Autodesk Fusion 360 part; units mm, degrees
note: some values were not read from the file. Set by a fixed rule: which sketch regions a step uses.
(part 5 of 6)
  spline S21 degree 5 poles (-7.8946, -5.2845) (-7.8923, -5.2844) (-7.8878, -5.2843) (-7.8811, -5.2842) (-7.8721, -5.284) (-7.8608, -5.2837) (-7.8496, -5.2835) (-7.8385, -5.2832) (-7.8273, -5.2828) (-7.8162, -5.2825) (-7.8052, -5.2821) (-7.7941, -5.2817) (-7.7831, -5.2813) (-7.7721, -5.2808) (-7.7611, -5.2803) (-7.7502, -5.2798) (-7.7393, -5.2793) (-7.7284, -5.2788) (-7.7175, -5.2782) (-7.7067, -5.2776) (-7.6959, -5.277) (-7.6852, -5.2764) (-7.6744, -5.2757) (-7.6637, -5.275) (-7.6531, -5.2743) (-7.6424, -5.2736) (-7.6318, -5.2729) (-7.6212, -5.2721) (-7.6107, -5.2713) (-7.6002, -5.2705) (-7.5897, -5.2697) (-7.5792, -5.2688) (-7.5688, -5.2679) (-7.5584, -5.2671) (-7.5481, -5.2661) (-7.5377, -5.2652) (-7.5274, -5.2642) (-7.5172, -5.2633) (-7.5069, -5.2623) (-7.4967, -5.2613) (-7.4865, -5.2602) (-7.4764, -5.2592) (-7.4663, -5.2581) (-7.4562, -5.257) (-7.4462, -5.2559) (-7.4362, -5.2547) (-7.4262, -5.2536) (-7.4163, -5.2524) (-7.4064, -5.2512) (-7.3965, -5.25) (-7.3866, -5.2487) (-7.3768, -5.2475) (-7.3671, -5.2462) (-7.3573, -5.2449) (-7.3476, -5.2436) (-7.3379, -5.2423) (-7.3283, -5.2409) (-7.3187, -5.2396) (-7.3091, -5.2382) (-7.2996, -5.2368) (-7.2901, -5.2354) (-7.2806, -5.2339) (-7.2712, -5.2325) (-7.2618, -5.231) (-7.2524, -5.2295) (-7.2431, -5.228) (-7.2338, -5.2265) (-7.2246, -5.225) (-7.2154, -5.2234) (-7.2062, -5.2219) (-7.197, -5.2203) (-7.1879, -5.2187) (-7.1789, -5.2171) (-7.1698, -5.2154) (-7.1608, -5.2138) (-7.1519, -5.2121) (-7.1429, -5.2104) (-7.1341, -5.2087) (-7.1252, -5.207) (-7.1164, -5.2053) (-7.1076, -5.2036) (-7.0989, -5.2018) (-7.0902, -5.2001) (-7.0815, -5.1983) (-7.0729, -5.1965) (-7.0643, -5.1947) (-7.0558, -5.1929) (-7.0473, -5.191) (-7.0388, -5.1892) (-7.0304, -5.1873) (-7.022, -5.1854) (-7.0136, -5.1836) (-7.0053, -5.1817) (-6.997, -5.1797) (-6.9888, -5.1778) (-6.9806, -5.1759) (-6.9725, -5.1739) (-6.9644, -5.172) (-6.9563, -5.17) (-6.9483, -5.168) (-6.9403, -5.166) (-6.9323, -5.164) (-6.9244, -5.162) (-6.9165, -5.16) (-6.9087, -5.158) (-6.9009, -5.1559) (-6.8932, -5.1539) (-6.8855, -5.1518) (-6.8778, -5.1498) (-6.8702, -5.1477) (-6.8626, -5.1456) (-6.8551, -5.1435) (-6.8476, -5.1414) (-6.8401, -5.1393) (-6.8327, -5.1371) (-6.8254, -5.135) (-6.818, -5.1329) (-6.8108, -5.1307) (-6.8035, -5.1286) (-6.7963, -5.1264) (-6.7892, -5.1242) (-6.7821, -5.1221) (-6.775, -5.1199) (-6.768, -5.1177) (-6.761, -5.1155) (-6.7541, -5.1133) (-6.7472, -5.1111) (-6.7404, -5.1089) (-6.7336, -5.1067) (-6.7269, -5.1045) (-6.7201, -5.1023) (-6.7135, -5.1) (-6.7069, -5.0978) (-6.7003, -5.0956) (-6.6938, -5.0933) (-6.6873, -5.0911) (-6.6809, -5.0889) (-6.6745, -5.0866) (-6.6682, -5.0844) (-6.6619, -5.0821) (-6.6556, -5.0799) (-6.6495, -5.0776) (-6.6433, -5.0754) (-6.6372, -5.0731) (-6.6312, -5.0709) (-6.6252, -5.0686) (-6.6192, -5.0664) (-6.6133, -5.0641) (-6.6074, -5.0618) (-6.6016, -5.0596) (-6.5959, -5.0573) (-6.5901, -5.0551) (-6.5845, -5.0528) (-6.5789, -5.0506) (-6.5733, -5.0483) (-6.5678, -5.0461) (-6.5623, -5.0439) (-6.5569, -5.0416) (-6.5515, -5.0394) (-6.5462, -5.0372) (-6.541, -5.0349) (-6.5357, -5.0327) (-6.5306, -5.0305) (-6.5255, -5.0283) (-6.5204, -5.0261) (-6.5154, -5.0239) (-6.5104, -5.0217) (-6.5055, -5.0195) (-6.5007, -5.0174) (-6.4959, -5.0152) (-6.4911, -5.013) (-6.4864, -5.0109) (-6.4818, -5.0087) (-6.4772, -5.0066) (-6.4727, -5.0045) (-6.4682, -5.0023) (-6.4637, -5.0002) (-6.4594, -4.9981) (-6.455, -4.9961) (-6.4508, -4.994) (-6.4466, -4.9919) (-6.4424, -4.9899) (-6.4383, -4.9878) (-6.4343, -4.9858) (-6.4303, -4.9838) (-6.4263, -4.9818) (-6.4224, -4.9798) (-6.4186, -4.9778) (-6.4149, -4.9759) (-6.4111, -4.9739) (-6.4075, -4.972) (-6.4039, -4.9701) (-6.4003, -4.9682) (-6.3969, -4.9664) (-6.3934, -4.9645) (-6.3901, -4.9627) (-6.3868, -4.9608) (-6.3835, -4.9591) (-6.3803, -4.9573) (-6.3772, -4.9555) (-6.3741, -4.9538) (-6.3711, -4.9521) (-6.3681, -4.9504) (-6.3652, -4.9487) (-6.3624, -4.9471) (-6.3596, -4.9454) (-6.3569, -4.9439) (-6.3543, -4.9423) (-6.3517, -4.9407) (-6.3491, -4.9392) (-6.3467, -4.9377) (-6.3443, -4.9363) (-6.3419, -4.9348) (-6.3396, -4.9334) (-6.3374, -4.932) (-6.3353, -4.9307) (-6.3332, -4.9294) (-6.3311, -4.9281) (-6.3292, -4.9268) (-6.3273, -4.9256) (-6.3254, -4.9244) (-6.3237, -4.9233) (-6.322, -4.9221) (-6.3203, -4.9211) (-6.3188, -4.92) (-6.3173, -4.919) (-6.3158, -4.918) (-6.3144, -4.9171) (-6.3131, -4.9162) (-6.3119, -4.9153) (-6.3107, -4.9145) (-6.3096, -4.9138) (-6.3086, -4.913) (-6.3076, -4.9124) (-6.3067, -4.9117) (-6.3059, -4.9111) (-6.3052, -4.9106) (-6.3045, -4.9101) (-6.3039, -4.9096) (-6.3033, -4.9092) (-6.3029, -4.9089) (-6.3026, -4.9086) (-6.3024, -4.9085) (-6.3022, -4.9084) (-6.3022, -4.9084) knots -1 -1 -1 -1 -1 -1 -0.99583333 -0.99166667 -0.9875 -0.98333333 -0.97916667 -0.975 -0.97083333 -0.96666667 -0.9625 -0.95833333 -0.95416667 -0.95 -0.94583333 -0.94166667 -0.9375 -0.93333333 -0.92916667 -0.925 -0.92083333 -0.91666667 -0.9125 -0.90833333 -0.90416667 -0.9 -0.89583333 -0.89166667 -0.8875 -0.88333333 -0.87916667 -0.875 -0.87083333 -0.86666667 -0.8625 -0.85833333 -0.85416667 -0.85 -0.84583333 -0.84166667 -0.8375 -0.83333333 -0.82916667 -0.825 -0.82083333 -0.81666667 -0.8125 -0.80833333 -0.80416667 -0.8 -0.79583333 -0.79166667 -0.7875 -0.78333333 -0.77916667 -0.775 -0.77083333 -0.76666667 -0.7625 -0.75833333 -0.75416667 -0.75 -0.74583333 -0.74166667 -0.7375 -0.73333333 -0.72916667 -0.725 -0.72083333 -0.71666667 -0.7125 -0.70833333 -0.70416667 -0.7 -0.69583333 -0.69166667 -0.6875 -0.68333333 -0.67916667 -0.675 -0.67083333 -0.66666667 -0.6625 -0.65833333 -0.65416667 -0.65 -0.64583333 -0.64166667 -0.6375 -0.63333333 -0.62916667 -0.625 -0.62083333 -0.61666667 -0.6125 -0.60833333 -0.60416667 -0.6 -0.59583333 -0.59166667 -0.5875 -0.58333333 -0.57916667 -0.575 -0.57083333 -0.56666667 -0.5625 -0.55833333 -0.55416667 -0.55 -0.54583333 -0.54166667 -0.5375 -0.53333333 -0.52916667 -0.525 -0.52083333 -0.51666667 -0.5125 -0.50833333 -0.50416667 -0.5 -0.49583333 -0.49166667 -0.4875 -0.48333333 -0.47916667 -0.475 -0.47083333 -0.46666667 -0.4625 -0.45833333 -0.45416667 -0.45 -0.44583333 -0.44166667 -0.4375 -0.43333333 -0.42916667 -0.425 -0.42083333 -0.41666667 -0.4125 -0.40833333 -0.40416667 -0.4 -0.39583333 -0.39166667 -0.3875 -0.38333333 -0.37916667 -0.375 -0.37083333 -0.36666667 -0.3625 -0.35833333 -0.35416667 -0.35 -0.34583333 -0.34166667 -0.3375 -0.33333333 -0.32916667 -0.325 -0.32083333 -0.31666667 -0.3125 -0.30833333 -0.30416667 -0.3 -0.29583333 -0.29166667 -0.2875 -0.28333333 -0.27916667 -0.275 -0.27083333 -0.26666667 -0.2625 -0.25833333 -0.25416667 -0.25 -0.24583333 -0.24166667 -0.2375 -0.23333333 -0.22916667 -0.225 -0.22083333 -0.21666667 -0.2125 -0.20833333 -0.20416667 -0.2 -0.19583333 -0.19166667 -0.1875 -0.18333333 -0.17916667 -0.175 -0.17083333 -0.16666667 -0.1625 -0.15833333 -0.15416667 -0.15 -0.14583333 -0.14166667 -0.1375 -0.13333333 -0.12916667 -0.125 -0.12083333 -0.11666667 -0.1125 -0.10833333 -0.10416667 -0.1 -0.09583333 -0.09166667 -0.0875 -0.08333333 -0.07916667 -0.075 -0.07083333 -0.06666667 -0.0625 -0.05833333 -0.05416667 -0.05 -0.04583333 -0.04166667 -0.0375 -0.03333333 -0.02916667 -0.025 -0.02083333 -0.01666667 -0.0125 -0.00833333 -0.00416667 0 0 0 0 0 0
  line L42 (-6.3022, -4.9084) -> (-6.3016, -4.9079)
  line L43 (-6.3016, -4.9079) -> (-5.7199, -4.4548)
  arc A22 (-5.7199, -4.4548) -> (-4.9636, -5.2844) centre (0, 0) ccw
  line L44 (-4.9636, -5.2844) -> (-5.4684, -5.8219)
  line L45 (-5.4684, -5.8219) -> (-5.4689, -5.8224)
  spline S22 degree 5 poles (-5.4689, -5.8224) (-5.469, -5.8225) (-5.4691, -5.8226) (-5.4692, -5.8228) (-5.4695, -5.823) (-5.4699, -5.8235) (-5.4703, -5.824) (-5.4708, -5.8245) (-5.4714, -5.8252) (-5.472, -5.8259) (-5.4727, -5.8266) (-5.4734, -5.8275) (-5.4742, -5.8284) (-5.475, -5.8293) (-5.4758, -5.8304) (-5.4768, -5.8314) (-5.4777, -5.8326) (-5.4787, -5.8338) (-5.4798, -5.8351) (-5.4809, -5.8364) (-5.482, -5.8378) (-5.4832, -5.8393) (-5.4845, -5.8408) (-5.4857, -5.8424) (-5.487, -5.8441) (-5.4884, -5.8458) (-5.4898, -5.8476) (-5.4912, -5.8494) (-5.4927, -5.8513) (-5.4942, -5.8533) (-5.4957, -5.8553) (-5.4973, -5.8574) (-5.4989, -5.8595) (-5.5006, -5.8617) (-5.5023, -5.864) (-5.504, -5.8663) (-5.5057, -5.8687) (-5.5075, -5.8711) (-5.5093, -5.8736) (-5.5111, -5.8762) (-5.513, -5.8788) (-5.5149, -5.8815) (-5.5168, -5.8842) (-5.5188, -5.887) (-5.5208, -5.8898) (-5.5228, -5.8927) (-5.5248, -5.8957) (-5.5269, -5.8987) (-5.529, -5.9018) (-5.5311, -5.9049) (-5.5332, -5.9081) (-5.5354, -5.9113) (-5.5376, -5.9146) (-5.5398, -5.918) (-5.542, -5.9214) (-5.5443, -5.9249) (-5.5465, -5.9284) (-5.5488, -5.9319) (-5.5511, -5.9356) (-5.5535, -5.9393) (-5.5558, -5.943) (-5.5582, -5.9468) (-5.5606, -5.9506) (-5.563, -5.9545) (-5.5654, -5.9585) (-5.5679, -5.9625) (-5.5703, -5.9665) (-5.5728, -5.9706) (-5.5753, -5.9748) (-5.5778, -5.979) (-5.5803, -5.9833) (-5.5829, -5.9876) (-5.5854, -5.992) (-5.588, -5.9964) (-5.5906, -6.0009) (-5.5932, -6.0054) (-5.5958, -6.01) (-5.5984, -6.0146) (-5.601, -6.0193) (-5.6036, -6.0241) (-5.6063, -6.0288) (-5.6089, -6.0337) (-5.6116, -6.0386) (-5.6143, -6.0435) (-5.617, -6.0485) (-5.6197, -6.0535) (-5.6224, -6.0586) (-5.6251, -6.0637) (-5.6278, -6.0689) (-5.6306, -6.0742) (-5.6333, -6.0795) (-5.6361, -6.0848) (-5.6388, -6.0902) (-5.6416, -6.0956) (-5.6444, -6.1011) (-5.6471, -6.1066) (-5.6499, -6.1122) (-5.6527, -6.1178) (-5.6555, -6.1235) (-5.6583, -6.1292) (-5.6611, -6.135) (-5.6639, -6.1408) (-5.6667, -6.1467) (-5.6695, -6.1526) (-5.6723, -6.1585) (-5.6751, -6.1645) (-5.6779, -6.1706) (-5.6808, -6.1767) (-5.6836, -6.1829) (-5.6864, -6.189) (-5.6892, -6.1953) (-5.6921, -6.2016) (-5.6949, -6.2079) (-5.6977, -6.2143) (-5.7006, -6.2207) (-5.7034, -6.2272) (-5.7062, -6.2337) (-5.709, -6.2402) (-5.7119, -6.2469) (-5.7147, -6.2535) (-5.7175, -6.2602) (-5.7204, -6.2669) (-5.7232, -6.2737) (-5.726, -6.2806) (-5.7288, -6.2874) (-5.7316, -6.2943) (-5.7344, -6.3013) (-5.7373, -6.3083) (-5.7401, -6.3154) (-5.7429, -6.3225) (-5.7457, -6.3296) (-5.7485, -6.3368) (-5.7513, -6.344) (-5.7541, -6.3513) (-5.7568, -6.3586) (-5.7596, -6.3659) (-5.7624, -6.3733) (-5.7652, -6.3808) (-5.7679, -6.3882) (-5.7707, -6.3958) (-5.7734, -6.4033) (-5.7762, -6.4109) (-5.7789, -6.4186) (-5.7817, -6.4263) (-5.7844, -6.434) (-5.7871, -6.4418) (-5.7898, -6.4496) (-5.7925, -6.4574) (-5.7952, -6.4653) (-5.7979, -6.4733) (-5.8006, -6.4813) (-5.8033, -6.4893) (-5.8059, -6.4973) (-5.8086, -6.5054) (-5.8112, -6.5136) (-5.8139, -6.5218) (-5.8165, -6.53) (-5.8191, -6.5382) (-5.8217, -6.5465) (-5.8243, -6.5549) (-5.8269, -6.5633) (-5.8295, -6.5717) (-5.8321, -6.5801) (-5.8346, -6.5886) (-5.8372, -6.5972) (-5.8397, -6.6057) (-5.8423, -6.6144) (-5.8448, -6.623) (-5.8473, -6.6317) (-5.8498, -6.6404) (-5.8523, -6.6492) (-5.8547, -6.658) (-5.8572, -6.6669) (-5.8596, -6.6757) (-5.8621, -6.6847) (-5.8645, -6.6936) (-5.8669, -6.7026) (-5.8693, -6.7117) (-5.8717, -6.7207) (-5.874, -6.7298) (-5.8764, -6.739) (-5.8787, -6.7482) (-5.8811, -6.7574) (-5.8834, -6.7666) (-5.8857, -6.7759) (-5.888, -6.7853) (-5.8902, -6.7946) (-5.8925, -6.804) (-5.8948, -6.8135) (-5.897, -6.8229) (-5.8992, -6.8324) (-5.9014, -6.842) (-5.9036, -6.8516) (-5.9057, -6.8612) (-5.9079, -6.8708) (-5.91, -6.8805) (-5.9122, -6.8902) (-5.9143, -6.9) (-5.9164, -6.9098) (-5.9184, -6.9196) (-5.9205, -6.9295) (-5.9225, -6.9394) (-5.9245, -6.9493) (-5.9266, -6.9593) (-5.9285, -6.9693) (-5.9305, -6.9793) (-5.9325, -6.9894) (-5.9344, -6.9995) (-5.9363, -7.0096) (-5.9382, -7.0198) (-5.9401, -7.03) (-5.942, -7.0402) (-5.9438, -7.0505) (-5.9457, -7.0608) (-5.9475, -7.0711) (-5.9493, -7.0815) (-5.9511, -7.0919) (-5.9528, -7.1023) (-5.9546, -7.1128) (-5.9563, -7.1232) (-5.958, -7.1338) (-5.9597, -7.1443) (-5.9613, -7.1549) (-5.963, -7.1656) (-5.9646, -7.1762) (-5.9662, -7.1869) (-5.9678, -7.1976) (-5.9693, -7.2084) (-5.9709, -7.2191) (-5.9724, -7.23) (-5.9739, -7.2408) (-5.9754, -7.2517) (-5.9769, -7.2626) (-5.9783, -7.2735) (-5.9797, -7.2845) (-5.9811, -7.2955) (-5.9825, -7.3065) (-5.9839, -7.3176) (-5.9852, -7.3287) (-5.9865, -7.3398) (-5.9878, -7.3509) (-5.9888, -7.3599) (-5.9896, -7.3666) (-5.9901, -7.3711) (-5.9903, -7.3733) knots 0 0 0 0 0 0 0.00416667 0.00833333 0.0125 0.01666667 0.02083333 0.025 0.02916667 0.03333333 0.0375 0.04166667 0.04583333 0.05 0.05416667 0.05833333 0.0625 0.06666667 0.07083333 0.075 0.07916667 0.08333333 0.0875 0.09166667 0.09583333 0.1 0.10416667 0.10833333 0.1125 0.11666667 0.12083333 0.125 0.12916667 0.13333333 0.1375 0.14166667 0.14583333 0.15 0.15416667 0.15833333 0.1625 0.16666667 0.17083333 0.175 0.17916667 0.18333333 0.1875 0.19166667 0.19583333 0.2 0.20416667 0.20833333 0.2125 0.21666667 0.22083333 0.225 0.22916667 0.23333333 0.2375 0.24166667 0.24583333 0.25 0.25416667 0.25833333 0.2625 0.26666667 0.27083333 0.275 0.27916667 0.28333333 0.2875 0.29166667 0.29583333 0.3 0.30416667 0.30833333 0.3125 0.31666667 0.32083333 0.325 0.32916667 0.33333333 0.3375 0.34166667 0.34583333 0.35 0.35416667 0.35833333 0.3625 0.36666667 0.37083333 0.375 0.37916667 0.38333333 0.3875 0.39166667 0.39583333 0.4 0.40416667 0.40833333 0.4125 0.41666667 0.42083333 0.425 0.42916667 0.43333333 0.4375 0.44166667 0.44583333 0.45 0.45416667 0.45833333 0.4625 0.46666667 0.47083333 0.475 0.47916667 0.48333333 0.4875 0.49166667 0.49583333 0.5 0.50416667 0.50833333 0.5125 0.51666667 0.52083333 0.525 0.52916667 0.53333333 0.5375 0.54166667 0.54583333 0.55 0.55416667 0.55833333 0.5625 0.56666667 0.57083333 0.575 0.57916667 0.58333333 0.5875 0.59166667 0.59583333 0.6 0.60416667 0.60833333 0.6125 0.61666667 0.62083333 0.625 0.62916667 0.63333333 0.6375 0.64166667 0.64583333 0.65 0.65416667 0.65833333 0.6625 0.66666667 0.67083333 0.675 0.67916667 0.68333333 0.6875 0.69166667 0.69583333 0.7 0.70416667 0.70833333 0.7125 0.71666667 0.72083333 0.725 0.72916667 0.73333333 0.7375 0.74166667 0.74583333 0.75 0.75416667 0.75833333 0.7625 0.76666667 0.77083333 0.775 0.77916667 0.78333333 0.7875 0.79166667 0.79583333 0.8 0.80416667 0.80833333 0.8125 0.81666667 0.82083333 0.825 0.82916667 0.83333333 0.8375 0.84166667 0.84583333 0.85 0.85416667 0.85833333 0.8625 0.86666667 0.87083333 0.875 0.87916667 0.88333333 0.8875 0.89166667 0.89583333 0.9 0.90416667 0.90833333 0.9125 0.91666667 0.92083333 0.925 0.92916667 0.93333333 0.9375 0.94166667 0.94583333 0.95 0.95416667 0.95833333 0.9625 0.96666667 0.97083333 0.975 0.97916667 0.98333333 0.9875 0.99166667 0.99583333 1 1 1 1 1 1
  arc A23 (-5.9903, -7.3733) -> (-5.4525, -7.7795) centre (0, 0) ccw
  spline S23 degree 5 poles (-5.4525, -7.7795) (-5.4504, -7.7786) (-5.4463, -7.7769) (-5.44, -7.7743) (-5.4317, -7.7709) (-5.4213, -7.7666) (-5.411, -7.7623) (-5.4007, -7.758) (-5.3904, -7.7536) (-5.3802, -7.7493) (-5.37, -7.7449) (-5.3598, -7.7406) (-5.3497, -7.7362) (-5.3396, -7.7318) (-5.3296, -7.7274) (-5.3195, -7.723) (-5.3096, -7.7186) (-5.2996, -7.7141) (-5.2897, -7.7097) (-5.2798, -7.7052) (-5.27, -7.7008) (-5.2602, -7.6963) (-5.2504, -7.6918) (-5.2407, -7.6873) (-5.231, -7.6828) (-5.2213, -7.6783) (-5.2117, -7.6737) (-5.2021, -7.6692) (-5.1925, -7.6647) (-5.183, -7.6601) (-5.1736, -7.6555) (-5.1641, -7.651) (-5.1547, -7.6464) (-5.1453, -7.6418) (-5.136, -7.6372) (-5.1267, -7.6326) (-5.1175, -7.628) (-5.1082, -7.6234) (-5.099, -7.6187) (-5.0899, -7.6141) (-5.0808, -7.6095) (-5.0717, -7.6048) (-5.0627, -7.6001) (-5.0537, -7.5955) (-5.0447, -7.5908) (-5.0358, -7.5861) (-5.0269, -7.5815) (-5.0181, -7.5768) (-5.0093, -7.5721) (-5.0005, -7.5674) (-4.9918, -7.5627) (-4.9831, -7.5579) (-4.9744, -7.5532) (-4.9658, -7.5485) (-4.9572, -7.5438) (-4.9487, -7.5391) (-4.9402, -7.5343) (-4.9317, -7.5296) (-4.9233, -7.5248) (-4.9149, -7.5201) (-4.9066, -7.5153) (-4.8983, -7.5106) (-4.89, -7.5058) (-4.8818, -7.501) (-4.8736, -7.4963) (-4.8654, -7.4915) (-4.8573, -7.4867) (-4.8492, -7.482) (-4.8412, -7.4772) (-4.8332, -7.4724) (-4.8253, -7.4676) (-4.8173, -7.4628) (-4.8095, -7.4581) (-4.8016, -7.4533) (-4.7938, -7.4485) (-4.7861, -7.4437) (-4.7784, -7.4389) (-4.7707, -7.4341) (-4.7631, -7.4293) (-4.7555, -7.4245) (-4.7479, -7.4198) (-4.7404, -7.415) (-4.7329, -7.4102) (-4.7255, -7.4054) (-4.7181, -7.4006) (-4.7107, -7.3958) (-4.7034, -7.391) (-4.6962, -7.3862) (-4.6889, -7.3815) (-4.6817, -7.3767) (-4.6746, -7.3719) (-4.6675, -7.3671) (-4.6604, -7.3624) (-4.6534, -7.3576) (-4.6464, -7.3528) (-4.6395, -7.3481) (-4.6326, -7.3433) (-4.6257, -7.3386) (-4.6189, -7.3338) (-4.6121, -7.3291) (-4.6054, -7.3243) (-4.5987, -7.3196) (-4.5921, -7.3148) (-4.5855, -7.3101) (-4.5789, -7.3054) (-4.5724, -7.3007) (-4.5659, -7.296) (-4.5595, -7.2913) (-4.5531, -7.2866) (-4.5467, -7.2819) (-4.5404, -7.2772) (-4.5341, -7.2725) (-4.5279, -7.2678) (-4.5217, -7.2632) (-4.5156, -7.2585) (-4.5095, -7.2539) (-4.5034, -7.2492) (-4.4974, -7.2446) (-4.4914, -7.24) (-4.4855, -7.2354) (-4.4796, -7.2308) (-4.4738, -7.2262) (-4.468, -7.2216) (-4.4623, -7.217) (-4.4565, -7.2124) (-4.4509, -7.2079) (-4.4453, -7.2034) (-4.4397, -7.1988) (-4.4341, -7.1943) (-4.4286, -7.1898) (-4.4232, -7.1853) (-4.4178, -7.1808) (-4.4124, -7.1764) (-4.4071, -7.1719) (-4.4018, -7.1675) (-4.3966, -7.1631) (-4.3914, -7.1586) (-4.3863, -7.1542) (-4.3812, -7.1499) (-4.3762, -7.1455) (-4.3711, -7.1411) (-4.3662, -7.1368) (-4.3613, -7.1325) (-4.3564, -7.1282) (-4.3516, -7.1239) (-4.3468, -7.1196) (-4.342, -7.1154) (-4.3373, -7.1111) (-4.3327, -7.1069) (-4.3281, -7.1027) (-4.3235, -7.0985) (-4.319, -7.0944) (-4.3145, -7.0902) (-4.3101, -7.0861) (-4.3057, -7.082) (-4.3014, -7.0779) (-4.2971, -7.0738) (-4.2929, -7.0698) (-4.2887, -7.0658) (-4.2845, -7.0618) (-4.2804, -7.0578) (-4.2764, -7.0539) (-4.2724, -7.0499) (-4.2684, -7.046) (-4.2645, -7.0421) (-4.2606, -7.0383) (-4.2568, -7.0344) (-4.253, -7.0306) (-4.2492, -7.0269) (-4.2455, -7.0231) (-4.2419, -7.0194) (-4.2383, -7.0157) (-4.2347, -7.012) (-4.2312, -7.0083) (-4.2278, -7.0047) (-4.2243, -7.0011) (-4.221, -6.9976) (-4.2176, -6.994) (-4.2144, -6.9905) (-4.2111, -6.987) (-4.208, -6.9836) (-4.2048, -6.9802) (-4.2017, -6.9768) (-4.1987, -6.9734) (-4.1957, -6.9701) (-4.1927, -6.9668) (-4.1898, -6.9636) (-4.187, -6.9604) (-4.1842, -6.9572) (-4.1814, -6.954) (-4.1787, -6.9509) (-4.176, -6.9478) (-4.1734, -6.9448) (-4.1708, -6.9418) (-4.1683, -6.9388) (-4.1658, -6.9359) (-4.1634, -6.933) (-4.161, -6.9302) (-4.1587, -6.9274) (-4.1564, -6.9246) (-4.1542, -6.9219) (-4.152, -6.9192) (-4.1498, -6.9165) (-4.1477, -6.9139) (-4.1457, -6.9114) (-4.1437, -6.9089) (-4.1417, -6.9064) (-4.1398, -6.904) (-4.138, -6.9016) (-4.1361, -6.8993) (-4.1344, -6.897) (-4.1327, -6.8947) (-4.131, -6.8925) (-4.1294, -6.8904) (-4.1278, -6.8883) (-4.1263, -6.8863) (-4.1248, -6.8843) (-4.1234, -6.8824) (-4.122, -6.8805) (-4.1207, -6.8787) (-4.1194, -6.8769) (-4.1182, -6.8752) (-4.117, -6.8735) (-4.1158, -6.8719) (-4.1148, -6.8704) (-4.1137, -6.8689) (-4.1127, -6.8675) (-4.1118, -6.8661) (-4.1109, -6.8648) (-4.11, -6.8635) (-4.1092, -6.8624) (-4.1085, -6.8612) (-4.1078, -6.8602) (-4.1072, -6.8592) (-4.1065, -6.8583) (-4.106, -6.8574) (-4.1055, -6.8567) (-4.105, -6.856) (-4.1046, -6.8553) (-4.1043, -6.8548) (-4.104, -6.8543) (-4.1037, -6.8539) (-4.1036, -6.8537) (-4.1035, -6.8536) (-4.1035, -6.8535) knots -1 -1 -1 -1 -1 -1 -0.99583333 -0.99166667 -0.9875 -0.98333333 -0.97916667 -0.975 -0.97083333 -0.96666667 -0.9625 -0.95833333 -0.95416667 -0.95 -0.94583333 -0.94166667 -0.9375 -0.93333333 -0.92916667 -0.925 -0.92083333 -0.91666667 -0.9125 -0.90833333 -0.90416667 -0.9 -0.89583333 -0.89166667 -0.8875 -0.88333333 -0.87916667 -0.875 -0.87083333 -0.86666667 -0.8625 -0.85833333 -0.85416667 -0.85 -0.84583333 -0.84166667 -0.8375 -0.83333333 -0.82916667 -0.825 -0.82083333 -0.81666667 -0.8125 -0.80833333 -0.80416667 -0.8 -0.79583333 -0.79166667 -0.7875 -0.78333333 -0.77916667 -0.775 -0.77083333 -0.76666667 -0.7625 -0.75833333 -0.75416667 -0.75 -0.74583333 -0.74166667 -0.7375 -0.73333333 -0.72916667 -0.725 -0.72083333 -0.71666667 -0.7125 -0.70833333 -0.70416667 -0.7 -0.69583333 -0.69166667 -0.6875 -0.68333333 -0.67916667 -0.675 -0.67083333 -0.66666667 -0.6625 -0.65833333 -0.65416667 -0.65 -0.64583333 -0.64166667 -0.6375 -0.63333333 -0.62916667 -0.625 -0.62083333 -0.61666667 -0.6125 -0.60833333 -0.60416667 -0.6 -0.59583333 -0.59166667 -0.5875 -0.58333333 -0.57916667 -0.575 -0.57083333 -0.56666667 -0.5625 -0.55833333 -0.55416667 -0.55 -0.54583333 -0.54166667 -0.5375 -0.53333333 -0.52916667 -0.525 -0.52083333 -0.51666667 -0.5125 -0.50833333 -0.50416667 -0.5 -0.49583333 -0.49166667 -0.4875 -0.48333333 -0.47916667 -0.475 -0.47083333 -0.46666667 -0.4625 -0.45833333 -0.45416667 -0.45 -0.44583333 -0.44166667 -0.4375 -0.43333333 -0.42916667 -0.425 -0.42083333 -0.41666667 -0.4125 -0.40833333 -0.40416667 -0.4 -0.39583333 -0.39166667 -0.3875 -0.38333333 -0.37916667 -0.375 -0.37083333 -0.36666667 -0.3625 -0.35833333 -0.35416667 -0.35 -0.34583333 -0.34166667 -0.3375 -0.33333333 -0.32916667 -0.325 -0.32083333 -0.31666667 -0.3125 -0.30833333 -0.30416667 -0.3 -0.29583333 -0.29166667 -0.2875 -0.28333333 -0.27916667 -0.275 -0.27083333 -0.26666667 -0.2625 -0.25833333 -0.25416667 -0.25 -0.24583333 -0.24166667 -0.2375 -0.23333333 -0.22916667 -0.225 -0.22083333 -0.21666667 -0.2125 -0.20833333 -0.20416667 -0.2 -0.19583333 -0.19166667 -0.1875 -0.18333333 -0.17916667 -0.175 -0.17083333 -0.16666667 -0.1625 -0.15833333 -0.15416667 -0.15 -0.14583333 -0.14166667 -0.1375 -0.13333333 -0.12916667 -0.125 -0.12083333 -0.11666667 -0.1125 -0.10833333 -0.10416667 -0.1 -0.09583333 -0.09166667 -0.0875 -0.08333333 -0.07916667 -0.075 -0.07083333 -0.06666667 -0.0625 -0.05833333 -0.05416667 -0.05 -0.04583333 -0.04166667 -0.0375 -0.03333333 -0.02916667 -0.025 -0.02083333 -0.01666667 -0.0125 -0.00833333 -0.00416667 0 0 0 0 0 0
  line L46 (-4.1035, -6.8535) -> (-4.1031, -6.8529)
  line L47 (-4.1031, -6.8529) -> (-3.7243, -6.2203)
  arc A24 (-3.7243, -6.2203) -> (-2.7195, -6.7206) centre (0, 0) ccw
  line L48 (-2.7195, -6.7206) -> (-2.9961, -7.4042)
  line L49 (-2.9961, -7.4042) -> (-2.9963, -7.4048)
  spline S24 degree 5 poles (-2.9963, -7.4048) (-2.9963, -7.4049) (-2.9964, -7.405) (-2.9965, -7.4053) (-2.9966, -7.4056) (-2.9968, -7.4062) (-2.9971, -7.4068) (-2.9973, -7.4075) (-2.9976, -7.4083) (-2.9979, -7.4092) (-2.9983, -7.4101) (-2.9987, -7.4112) (-2.9991, -7.4123) (-2.9995, -7.4135) (-2.9999, -7.4147) (-3.0004, -7.4161) (-3.0008, -7.4175) (-3.0014, -7.419) (-3.0019, -7.4206) (-3.0024, -7.4222) (-3.003, -7.424) (-3.0036, -7.4258) (-3.0041, -7.4276) (-3.0048, -7.4296) (-3.0054, -7.4316) (-3.006, -7.4337) (-3.0067, -7.4359) (-3.0074, -7.4381) (-3.008, -7.4404) (-3.0087, -7.4428) (-3.0094, -7.4452) (-3.0102, -7.4477) (-3.0109, -7.4503) (-3.0116, -7.4529) (-3.0124, -7.4557) (-3.0131, -7.4584) (-3.0139, -7.4613) (-3.0147, -7.4642) (-3.0155, -7.4672) (-3.0163, -7.4702) (-3.0171, -7.4734) (-3.0179, -7.4765) (-3.0187, -7.4798) (-3.0195, -7.4831) (-3.0203, -7.4864) (-3.0211, -7.4899) (-3.022, -7.4934) (-3.0228, -7.4969) (-3.0237, -7.5006) (-3.0245, -7.5042) (-3.0253, -7.508) (-3.0262, -7.5118) (-3.027, -7.5156) (-3.0279, -7.5196) (-3.0287, -7.5235) (-3.0296, -7.5276) (-3.0304, -7.5317) (-3.0313, -7.5358) (-3.0321, -7.5401) (-3.033, -7.5443) (-3.0338, -7.5487) (-3.0346, -7.5531) (-3.0355, -7.5575) (-3.0363, -7.562) (-3.0372, -7.5666) (-3.038, -7.5712) (-3.0388, -7.5759) (-3.0396, -7.5806) (-3.0405, -7.5854) (-3.0413, -7.5902) (-3.0421, -7.5951) (-3.0429, -7.6001) (-3.0437, -7.6051) (-3.0445, -7.6101) (-3.0453, -7.6152) (-3.0461, -7.6204) (-3.0468, -7.6256) (-3.0476, -7.6308) (-3.0483, -7.6362) (-3.0491, -7.6415) (-3.0498, -7.647) (-3.0506, -7.6524) (-3.0513, -7.6579) (-3.052, -7.6635) (-3.0527, -7.6691) (-3.0534, -7.6748) (-3.0541, -7.6805) (-3.0548, -7.6863) (-3.0555, -7.6921) (-3.0561, -7.698) (-3.0568, -7.7039) (-3.0574, -7.7099) (-3.058, -7.7159) (-3.0586, -7.722) (-3.0592, -7.7281) (-3.0598, -7.7342) (-3.0604, -7.7404) (-3.061, -7.7467) (-3.0615, -7.753) (-3.0621, -7.7593) (-3.0626, -7.7657) (-3.0631, -7.7722) (-3.0636, -7.7786) (-3.0641, -7.7852) (-3.0645, -7.7917) (-3.065, -7.7984) (-3.0654, -7.805) (-3.0659, -7.8117) (-3.0663, -7.8185) (-3.0667, -7.8253) (-3.0671, -7.8321) (-3.0674, -7.839) (-3.0678, -7.8459) (-3.0681, -7.8529) (-3.0684, -7.8599) (-3.0687, -7.867) (-3.069, -7.8741) (-3.0693, -7.8812) (-3.0695, -7.8884) (-3.0698, -7.8956) (-3.07, -7.9029) (-3.0702, -7.9102) (-3.0704, -7.9175) (-3.0705, -7.9249) (-3.0707, -7.9323) (-3.0708, -7.9398) (-3.0709, -7.9473) (-3.071, -7.9549) (-3.0711, -7.9624) (-3.0711, -7.9701) (-3.0712, -7.9777) (-3.0712, -7.9854) (-3.0712, -7.9932) (-3.0712, -8.001) (-3.0711, -8.0088) (-3.071, -8.0167) (-3.071, -8.0246) (-3.0709, -8.0325) (-3.0707, -8.0405) (-3.0706, -8.0485) (-3.0704, -8.0565) (-3.0702, -8.0646) (-3.07, -8.0727) (-3.0698, -8.0809) (-3.0695, -8.0891) (-3.0693, -8.0973) (-3.069, -8.1056) (-3.0687, -8.1139) (-3.0683, -8.1222) (-3.068, -8.1306) (-3.0676, -8.139) (-3.0672, -8.1474) (-3.0668, -8.1559) (-3.0663, -8.1644) (-3.0658, -8.173) (-3.0653, -8.1816) (-3.0648, -8.1902) (-3.0643, -8.1988) (-3.0637, -8.2075) (-3.0631, -8.2162) (-3.0625, -8.225) (-3.0619, -8.2338) (-3.0612, -8.2426) (-3.0605, -8.2514) (-3.0598, -8.2603) (-3.0591, -8.2692) (-3.0584, -8.2782) (-3.0576, -8.2872) (-3.0568, -8.2962) (-3.0559, -8.3052) (-3.0551, -8.3143) (-3.0542, -8.3234) (-3.0533, -8.3325) (-3.0524, -8.3417) (-3.0514, -8.3509) (-3.0505, -8.3601) (-3.0495, -8.3694) (-3.0484, -8.3787) (-3.0474, -8.388) (-3.0463, -8.3973) (-3.0452, -8.4067) (-3.044, -8.4161) (-3.0429, -8.4256) (-3.0417, -8.435) (-3.0405, -8.4445) (-3.0393, -8.454) (-3.038, -8.4636) (-3.0367, -8.4732) (-3.0354, -8.4828) (-3.034, -8.4924) (-3.0327, -8.5021) (-3.0313, -8.5118) (-3.0299, -8.5215) (-3.0284, -8.5313) (-3.0269, -8.541) (-3.0254, -8.5508) (-3.0239, -8.5607) (-3.0223, -8.5705) (-3.0207, -8.5804) (-3.0191, -8.5903) (-3.0175, -8.6003) (-3.0158, -8.6102) (-3.0141, -8.6202) (-3.0124, -8.6302) (-3.0106, -8.6403) (-3.0088, -8.6503) (-3.007, -8.6604) (-3.0052, -8.6706) (-3.0033, -8.6807) (-3.0014, -8.6909) (-2.9995, -8.7011) (-2.9975, -8.7113) (-2.9955, -8.7215) (-2.9935, -8.7318) (-2.9915, -8.7421) (-2.9894, -8.7524) (-2.9873, -8.7627) (-2.9852, -8.7731) (-2.983, -8.7835) (-2.9808, -8.7939) (-2.9786, -8.8043) (-2.9764, -8.8148) (-2.9741, -8.8252) (-2.9718, -8.8357) (-2.9695, -8.8463) (-2.9671, -8.8568) (-2.9647, -8.8674) (-2.9623, -8.878) (-2.9598, -8.8886) (-2.9573, -8.8992) (-2.9548, -8.9099) (-2.9523, -8.9206) (-2.9497, -8.9312) (-2.9471, -8.942) (-2.9445, -8.9527) (-2.9418, -8.9635) (-2.9391, -8.9743) (-2.9364, -8.9851) (-2.9336, -8.9959) (-2.9308, -9.0067) (-2.928, -9.0176) (-2.9257, -9.0263) (-2.924, -9.0328) (-2.9228, -9.0372) (-2.9223, -9.0394) knots 0 0 0 0 0 0 0.00416667 0.00833333 0.0125 0.01666667 0.02083333 0.025 0.02916667 0.03333333 0.0375 0.04166667 0.04583333 0.05 0.05416667 0.05833333 0.0625 0.06666667 0.07083333 0.075 0.07916667 0.08333333 0.0875 0.09166667 0.09583333 0.1 0.10416667 0.10833333 0.1125 0.11666667 0.12083333 0.125 0.12916667 0.13333333 0.1375 0.14166667 0.14583333 0.15 0.15416667 0.15833333 0.1625 0.16666667 0.17083333 0.175 0.17916667 0.18333333 0.1875 0.19166667 0.19583333 0.2 0.20416667 0.20833333 0.2125 0.21666667 0.22083333 0.225 0.22916667 0.23333333 0.2375 0.24166667 0.24583333 0.25 0.25416667 0.25833333 0.2625 0.26666667 0.27083333 0.275 0.27916667 0.28333333 0.2875 0.29166667 0.29583333 0.3 0.30416667 0.30833333 0.3125 0.31666667 0.32083333 0.325 0.32916667 0.33333333 0.3375 0.34166667 0.34583333 0.35 0.35416667 0.35833333 0.3625 0.36666667 0.37083333 0.375 0.37916667 0.38333333 0.3875 0.39166667 0.39583333 0.4 0.40416667 0.40833333 0.4125 0.41666667 0.42083333 0.425 0.42916667 0.43333333 0.4375 0.44166667 0.44583333 0.45 0.45416667 0.45833333 0.4625 0.46666667 0.47083333 0.475 0.47916667 0.48333333 0.4875 0.49166667 0.49583333 0.5 0.50416667 0.50833333 0.5125 0.51666667 0.52083333 0.525 0.52916667 0.53333333 0.5375 0.54166667 0.54583333 0.55 0.55416667 0.55833333 0.5625 0.56666667 0.57083333 0.575 0.57916667 0.58333333 0.5875 0.59166667 0.59583333 0.6 0.60416667 0.60833333 0.6125 0.61666667 0.62083333 0.625 0.62916667 0.63333333 0.6375 0.64166667 0.64583333 0.65 0.65416667 0.65833333 0.6625 0.66666667 0.67083333 0.675 0.67916667 0.68333333 0.6875 0.69166667 0.69583333 0.7 0.70416667 0.70833333 0.7125 0.71666667 0.72083333 0.725 0.72916667 0.73333333 0.7375 0.74166667 0.74583333 0.75 0.75416667 0.75833333 0.7625 0.76666667 0.77083333 0.775 0.77916667 0.78333333 0.7875 0.79166667 0.79583333 0.8 0.80416667 0.80833333 0.8125 0.81666667 0.82083333 0.825 0.82916667 0.83333333 0.8375 0.84166667 0.84583333 0.85 0.85416667 0.85833333 0.8625 0.86666667 0.87083333 0.875 0.87916667 0.88333333 0.8875 0.89166667 0.89583333 0.9 0.90416667 0.90833333 0.9125 0.91666667 0.92083333 0.925 0.92916667 0.93333333 0.9375 0.94166667 0.94583333 0.95 0.95416667 0.95833333 0.9625 0.96666667 0.97083333 0.975 0.97916667 0.98333333 0.9875 0.99166667 0.99583333 1 1 1 1 1 1
  arc A25 (-2.9223, -9.0394) -> (-2.2741, -9.2238) centre (0, 0) ccw
  spline S25 degree 5 poles (-2.2741, -9.2238) (-2.2724, -9.2223) (-2.2691, -9.2192) (-2.2642, -9.2145) (-2.2577, -9.2083) (-2.2496, -9.2005) (-2.2415, -9.1928) (-2.2335, -9.185) (-2.2255, -9.1773) (-2.2175, -9.1696) (-2.2096, -9.1618) (-2.2017, -9.1541) (-2.1938, -9.1463) (-2.186, -9.1386) (-2.1782, -9.1308) (-2.1705, -9.1231) (-2.1627, -9.1154) (-2.1551, -9.1076) (-2.1474, -9.0999) (-2.1398, -9.0922) (-2.1323, -9.0845) (-2.1247, -9.0768) (-2.1173, -9.069) (-2.1098, -9.0613) (-2.1024, -9.0536) (-2.095, -9.0459) (-2.0877, -9.0382) (-2.0804, -9.0305) (-2.0731, -9.0228) (-2.0659, -9.0152) (-2.0587, -9.0075) (-2.0515, -8.9998) (-2.0444, -8.9921) (-2.0373, -8.9845) (-2.0303, -8.9768) (-2.0233, -8.9692) (-2.0163, -8.9615) (-2.0094, -8.9539) (-2.0025, -8.9462) (-1.9957, -8.9386) (-1.9888, -8.931) (-1.9821, -8.9234) (-1.9753, -8.9158) (-1.9686, -8.9082) (-1.962, -8.9006) (-1.9553, -8.893) (-1.9487, -8.8854) (-1.9422, -8.8779) (-1.9357, -8.8703) (-1.9292, -8.8628) (-1.9227, -8.8552) (-1.9163, -8.8477) (-1.91, -8.8401) (-1.9036, -8.8326) (-1.8973, -8.8251) (-1.8911, -8.8176) (-1.8849, -8.8101) (-1.8787, -8.8027) (-1.8726, -8.7952) (-1.8665, -8.7877) (-1.8604, -8.7803) (-1.8544, -8.7729) (-1.8484, -8.7654) (-1.8424, -8.758) (-1.8365, -8.7506) (-1.8306, -8.7432) (-1.8248, -8.7358) (-1.819, -8.7285) (-1.8132, -8.7211) (-1.8075, -8.7138) (-1.8018, -8.7064) (-1.7961, -8.6991) (-1.7905, -8.6918) (-1.785, -8.6845) (-1.7794, -8.6772) (-1.7739, -8.67) (-1.7684, -8.6627) (-1.763, -8.6555) (-1.7576, -8.6483) (-1.7523, -8.6411) (-1.747, -8.6339) (-1.7417, -8.6267) (-1.7365, -8.6195) (-1.7313, -8.6124) (-1.7261, -8.6052) (-1.721, -8.5981) (-1.7159, -8.591) (-1.7108, -8.5839) (-1.7058, -8.5769) (-1.7008, -8.5698) (-1.6959, -8.5628) (-1.691, -8.5557) (-1.6861, -8.5487) (-1.6813, -8.5418) (-1.6765, -8.5348) (-1.6718, -8.5278) (-1.6671, -8.5209) (-1.6624, -8.514) (-1.6577, -8.5071) (-1.6531, -8.5002) (-1.6486, -8.4934) (-1.644, -8.4865) (-1.6396, -8.4797) (-1.6351, -8.4729) (-1.6307, -8.4662) (-1.6263, -8.4594) (-1.622, -8.4527) (-1.6177, -8.446) (-1.6134, -8.4393) (-1.6092, -8.4326) (-1.605, -8.4259) (-1.6008, -8.4193) (-1.5967, -8.4127) (-1.5926, -8.4061) (-1.5886, -8.3996) (-1.5846, -8.393) (-1.5806, -8.3865) (-1.5767, -8.38) (-1.5728, -8.3736) (-1.5689, -8.3671) (-1.5651, -8.3607) (-1.5613, -8.3543) (-1.5576, -8.348) (-1.5538, -8.3416) (-1.5502, -8.3353) (-1.5465, -8.329) (-1.5429, -8.3227) (-1.5394, -8.3165) (-1.5358, -8.3103) (-1.5323, -8.3041) (-1.5289, -8.298) (-1.5255, -8.2918) (-1.5221, -8.2857) (-1.5187, -8.2796) (-1.5154, -8.2736) (-1.5121, -8.2676) (-1.5089, -8.2616) (-1.5057, -8.2556) (-1.5025, -8.2497) (-1.4994, -8.2438) (-1.4963, -8.238) (-1.4932, -8.2321) (-1.4902, -8.2263) (-1.4872, -8.2205) (-1.4843, -8.2148) (-1.4813, -8.2091) (-1.4785, -8.2034) (-1.4756, -8.1978) (-1.4728, -8.1921) (-1.47, -8.1866) (-1.4673, -8.181) (-1.4646, -8.1755) (-1.4619, -8.17) (-1.4593, -8.1646) (-1.4567, -8.1592) (-1.4541, -8.1538) (-1.4516, -8.1485) (-1.4491, -8.1432) (-1.4466, -8.1379) (-1.4442, -8.1327) (-1.4418, -8.1275) (-1.4394, -8.1223) (-1.4371, -8.1172) (-1.4348, -8.1121) (-1.4326, -8.1071) (-1.4304, -8.1021) (-1.4282, -8.0971) (-1.426, -8.0922) (-1.4239, -8.0873) (-1.4218, -8.0825) (-1.4198, -8.0777) (-1.4177, -8.073) (-1.4157, -8.0682) (-1.4138, -8.0636) (-1.4119, -8.0589) (-1.41, -8.0544) (-1.4081, -8.0498) (-1.4063, -8.0453) (-1.4045, -8.0409) (-1.4028, -8.0365) (-1.401, -8.0321) (-1.3994, -8.0278) (-1.3977, -8.0235) (-1.3961, -8.0193) (-1.3945, -8.0151) (-1.3929, -8.011) (-1.3914, -8.0069) (-1.3899, -8.0029) (-1.3884, -7.9989) (-1.387, -7.9949) (-1.3856, -7.9911) (-1.3842, -7.9872) (-1.3828, -7.9834) (-1.3815, -7.9797) (-1.3802, -7.976) (-1.379, -7.9724) (-1.3778, -7.9688) (-1.3766, -7.9653) (-1.3754, -7.9619) (-1.3743, -7.9585) (-1.3732, -7.9551) (-1.3721, -7.9518) (-1.3711, -7.9486) (-1.37, -7.9454) (-1.3691, -7.9423) (-1.3681, -7.9392) (-1.3672, -7.9362) (-1.3663, -7.9332) (-1.3654, -7.9303) (-1.3645, -7.9275) (-1.3637, -7.9247) (-1.3629, -7.922) (-1.3622, -7.9194) (-1.3614, -7.9168) (-1.3607, -7.9143) (-1.36, -7.9119) (-1.3594, -7.9095) (-1.3587, -7.9072) (-1.3581, -7.9049) (-1.3576, -7.9027) (-1.357, -7.9006) (-1.3565, -7.8986) (-1.356, -7.8966) (-1.3555, -7.8947) (-1.355, -7.8928) (-1.3546, -7.8911) (-1.3542, -7.8894) (-1.3538, -7.8878) (-1.3534, -7.8862) (-1.3531, -7.8848) (-1.3528, -7.8834) (-1.3525, -7.8821) (-1.3522, -7.8809) (-1.352, -7.8797) (-1.3517, -7.8786) (-1.3515, -7.8776) (-1.3513, -7.8767) (-1.3512, -7.8759) (-1.351, -7.8752) (-1.3509, -7.8745) (-1.3508, -7.8739) (-1.3507, -7.8735) (-1.3507, -7.8733) (-1.3506, -7.8731) (-1.3506, -7.8731) knots -1 -1 -1 -1 -1 -1 -0.99583333 -0.99166667 -0.9875 -0.98333333 -0.97916667 -0.975 -0.97083333 -0.96666667 -0.9625 -0.95833333 -0.95416667 -0.95 -0.94583333 -0.94166667 -0.9375 -0.93333333 -0.92916667 -0.925 -0.92083333 -0.91666667 -0.9125 -0.90833333 -0.90416667 -0.9 -0.89583333 -0.89166667 -0.8875 -0.88333333 -0.87916667 -0.875 -0.87083333 -0.86666667 -0.8625 -0.85833333 -0.85416667 -0.85 -0.84583333 -0.84166667 -0.8375 -0.83333333 -0.82916667 -0.825 -0.82083333 -0.81666667 -0.8125 -0.80833333 -0.80416667 -0.8 -0.79583333 -0.79166667 -0.7875 -0.78333333 -0.77916667 -0.775 -0.77083333 -0.76666667 -0.7625 -0.75833333 -0.75416667 -0.75 -0.74583333 -0.74166667 -0.7375 -0.73333333 -0.72916667 -0.725 -0.72083333 -0.71666667 -0.7125 -0.70833333 -0.70416667 -0.7 -0.69583333 -0.69166667 -0.6875 -0.68333333 -0.67916667 -0.675 -0.67083333 -0.66666667 -0.6625 -0.65833333 -0.65416667 -0.65 -0.64583333 -0.64166667 -0.6375 -0.63333333 -0.62916667 -0.625 -0.62083333 -0.61666667 -0.6125 -0.60833333 -0.60416667 -0.6 -0.59583333 -0.59166667 -0.5875 -0.58333333 -0.57916667 -0.575 -0.57083333 -0.56666667 -0.5625 -0.55833333 -0.55416667 -0.55 -0.54583333 -0.54166667 -0.5375 -0.53333333 -0.52916667 -0.525 -0.52083333 -0.51666667 -0.5125 -0.50833333 -0.50416667 -0.5 -0.49583333 -0.49166667 -0.4875 -0.48333333 -0.47916667 -0.475 -0.47083333 -0.46666667 -0.4625 -0.45833333 -0.45416667 -0.45 -0.44583333 -0.44166667 -0.4375 -0.43333333 -0.42916667 -0.425 -0.42083333 -0.41666667 -0.4125 -0.40833333 -0.40416667 -0.4 -0.39583333 -0.39166667 -0.3875 -0.38333333 -0.37916667 -0.375 -0.37083333 -0.36666667 -0.3625 -0.35833333 -0.35416667 -0.35 -0.34583333 -0.34166667 -0.3375 -0.33333333 -0.32916667 -0.325 -0.32083333 -0.31666667 -0.3125 -0.30833333 -0.30416667 -0.3 -0.29583333 -0.29166667 -0.2875 -0.28333333 -0.27916667 -0.275 -0.27083333 -0.26666667 -0.2625 -0.25833333 -0.25416667 -0.25 -0.24583333 -0.24166667 -0.2375 -0.23333333 -0.22916667 -0.225 -0.22083333 -0.21666667 -0.2125 -0.20833333 -0.20416667 -0.2 -0.19583333 -0.19166667 -0.1875 -0.18333333 -0.17916667 -0.175 -0.17083333 -0.16666667 -0.1625 -0.15833333 -0.15416667 -0.15 -0.14583333 -0.14166667 -0.1375 -0.13333333 -0.12916667 -0.125 -0.12083333 -0.11666667 -0.1125 -0.10833333 -0.10416667 -0.1 -0.09583333 -0.09166667 -0.0875 -0.08333333 -0.07916667 -0.075 -0.07083333 -0.06666667 -0.0625 -0.05833333 -0.05416667 -0.05 -0.04583333 -0.04166667 -0.0375 -0.03333333 -0.02916667 -0.025 -0.02083333 -0.01666667 -0.0125 -0.00833333 -0.00416667 0 0 0 0 0 0
  line L50 (-1.3506, -7.8731) -> (-1.3505, -7.8724)
  line L51 (-1.3505, -7.8724) -> (-1.2258, -7.1456)
  arc A26 (-1.2258, -7.1456) -> (-0.1081, -7.2492) centre (0, 0) ccw
  line L52 (-0.1081, -7.2492) -> (-0.119, -7.9865)
  line L53 (-0.119, -7.9865) -> (-0.119, -7.9872)
  spline S26 degree 5 poles (-0.119, -7.9872) (-0.119, -7.9873) (-0.119, -7.9874) (-0.119, -7.9877) (-0.119, -7.9881) (-0.119, -7.9886) (-0.119, -7.9893) (-0.119, -7.9901) (-0.119, -7.9909) (-0.119, -7.9918) (-0.119, -7.9929) (-0.1189, -7.994) (-0.1189, -7.9951) (-0.1189, -7.9964) (-0.1188, -7.9977) (-0.1188, -7.9992) (-0.1187, -8.0007) (-0.1186, -8.0022) (-0.1185, -8.0039) (-0.1184, -8.0056) (-0.1183, -8.0074) (-0.1182, -8.0093) (-0.1181, -8.0113) (-0.118, -8.0133) (-0.1178, -8.0154) (-0.1177, -8.0176) (-0.1175, -8.0199) (-0.1173, -8.0222) (-0.1171, -8.0246) (-0.1169, -8.027) (-0.1167, -8.0296) (-0.1165, -8.0322) (-0.1162, -8.0349) (-0.1159, -8.0376) (-0.1157, -8.0404) (-0.1154, -8.0433) (-0.1151, -8.0462) (-0.1147, -8.0492) (-0.1144, -8.0523) (-0.114, -8.0554) (-0.1136, -8.0586) (-0.1132, -8.0618) (-0.1128, -8.0652) (-0.1124, -8.0685) (-0.112, -8.072) (-0.1115, -8.0755) (-0.111, -8.079) (-0.1105, -8.0826) (-0.11, -8.0863) (-0.1094, -8.0901) (-0.1088, -8.0939) (-0.1083, -8.0977) (-0.1077, -8.1016) (-0.107, -8.1056) (-0.1064, -8.1096) (-0.1057, -8.1137) (-0.105, -8.1178) (-0.1043, -8.122) (-0.1036, -8.1262) (-0.1028, -8.1305) (-0.102, -8.1349) (-0.1012, -8.1393) (-0.1004, -8.1437) (-0.0996, -8.1482) (-0.0987, -8.1528) (-0.0978, -8.1574) (-0.0969, -8.162) (-0.096, -8.1667) (-0.095, -8.1715) (-0.094, -8.1763) (-0.093, -8.1812) (-0.092, -8.1861) (-0.0909, -8.191) (-0.0898, -8.196) (-0.0887, -8.2011) (-0.0876, -8.2061) (-0.0864, -8.2113) (-0.0852, -8.2165) (-0.084, -8.2217) (-0.0828, -8.227) (-0.0815, -8.2323) (-0.0802, -8.2377) (-0.0789, -8.2431) (-0.0775, -8.2485) (-0.0762, -8.254) (-0.0748, -8.2596) (-0.0733, -8.2652) (-0.0719, -8.2708) (-0.0704, -8.2765) (-0.0689, -8.2822) (-0.0674, -8.2879) (-0.0658, -8.2937) (-0.0642, -8.2995) (-0.0626, -8.3054) (-0.061, -8.3113) (-0.0593, -8.3173) (-0.0576, -8.3233) (-0.0558, -8.3293) (-0.0541, -8.3354) (-0.0523, -8.3415) (-0.0505, -8.3477) (-0.0486, -8.3538) (-0.0467, -8.3601) (-0.0448, -8.3663) (-0.0429, -8.3726) (-0.0409, -8.379) (-0.0389, -8.3853) (-0.0369, -8.3917) (-0.0349, -8.3982) (-0.0328, -8.4047) (-0.0307, -8.4112) (-0.0285, -8.4177) (-0.0263, -8.4243) (-0.0241, -8.4309) (-0.0219, -8.4376) (-0.0196, -8.4443) (-0.0173, -8.451) (-0.015, -8.4578) (-0.0126, -8.4645) (-0.0103, -8.4714) (-0.0078, -8.4782) (-0.0054, -8.4851) (-0.0029, -8.492) (-0.0004, -8.499) (0.0022, -8.5059) (0.0047, -8.513) (0.0074, -8.52) (0.01, -8.5271) (0.0127, -8.5342) (0.0154, -8.5413) (0.0181, -8.5485) (0.0209, -8.5556) (0.0237, -8.5629) (0.0265, -8.5701) (0.0294, -8.5774) (0.0323, -8.5847) (0.0352, -8.592) (0.0382, -8.5994) (0.0412, -8.6068) (0.0442, -8.6142) (0.0473, -8.6216) (0.0504, -8.6291) (0.0535, -8.6366) (0.0567, -8.6441) (0.0598, -8.6517) (0.0631, -8.6593) (0.0663, -8.6669) (0.0696, -8.6745) (0.073, -8.6821) (0.0763, -8.6898) (0.0797, -8.6975) (0.0831, -8.7053) (0.0866, -8.713) (0.0901, -8.7208) (0.0936, -8.7286) (0.0972, -8.7364) (0.1008, -8.7443) (0.1044, -8.7521) (0.1081, -8.76) (0.1118, -8.7679) (0.1155, -8.7759) (0.1193, -8.7838) (0.1231, -8.7918) (0.1269, -8.7998) (0.1308, -8.8079) (0.1347, -8.8159) (0.1386, -8.824) (0.1426, -8.8321) (0.1466, -8.8402) (0.1506, -8.8483) (0.1547, -8.8565) (0.1588, -8.8646) (0.1629, -8.8728) (0.1671, -8.881) (0.1713, -8.8893) (0.1756, -8.8975) (0.1798, -8.9058) (0.1842, -8.9141) (0.1885, -8.9224) (0.1929, -8.9307) (0.1973, -8.9391) (0.2018, -8.9474) (0.2063, -8.9558) (0.2108, -8.9642) (0.2153, -8.9726) (0.2199, -8.9811) (0.2246, -8.9895) (0.2292, -8.998) (0.2339, -9.0065) (0.2387, -9.015) (0.2434, -9.0235) (0.2482, -9.032) (0.2531, -9.0406) (0.2579, -9.0492) (0.2629, -9.0577) (0.2678, -9.0663) (0.2728, -9.0749) (0.2778, -9.0836) (0.2829, -9.0922) (0.2879, -9.1009) (0.2931, -9.1095) (0.2982, -9.1182) (0.3034, -9.1269) (0.3086, -9.1357) (0.3139, -9.1444) (0.3192, -9.1531) (0.3246, -9.1619) (0.3299, -9.1707) (0.3353, -9.1794) (0.3408, -9.1882) (0.3463, -9.197) (0.3518, -9.2059) (0.3573, -9.2147) (0.3629, -9.2235) (0.3685, -9.2324) (0.3742, -9.2413) (0.3799, -9.2501) (0.3856, -9.259) (0.3914, -9.2679) (0.3972, -9.2769) (0.403, -9.2858) (0.4089, -9.2947) (0.4148, -9.3037) (0.4207, -9.3126) (0.4267, -9.3216) (0.4327, -9.3306) (0.4388, -9.3396) (0.4449, -9.3486) (0.451, -9.3576) (0.4571, -9.3666) (0.4633, -9.3756) (0.4696, -9.3847) (0.4758, -9.3937) (0.4821, -9.4028) (0.4885, -9.4118) (0.4948, -9.4209) (0.5012, -9.43) (0.5077, -9.4391) (0.5142, -9.4481) (0.5207, -9.4573) (0.5272, -9.4664) (0.5325, -9.4737) (0.5365, -9.4791) (0.5391, -9.4828) (0.5405, -9.4846) knots 0 0 0 0 0 0 0.00416667 0.00833333 0.0125 0.01666667 0.02083333 0.025 0.02916667 0.03333333 0.0375 0.04166667 0.04583333 0.05 0.05416667 0.05833333 0.0625 0.06666667 0.07083333 0.075 0.07916667 0.08333333 0.0875 0.09166667 0.09583333 0.1 0.10416667 0.10833333 0.1125 0.11666667 0.12083333 0.125 0.12916667 0.13333333 0.1375 0.14166667 0.14583333 0.15 0.15416667 0.15833333 0.1625 0.16666667 0.17083333 0.175 0.17916667 0.18333333 0.1875 0.19166667 0.19583333 0.2 0.20416667 0.20833333 0.2125 0.21666667 0.22083333 0.225 0.22916667 0.23333333 0.2375 0.24166667 0.24583333 0.25 0.25416667 0.25833333 0.2625 0.26666667 0.27083333 0.275 0.27916667 0.28333333 0.2875 0.29166667 0.29583333 0.3 0.30416667 0.30833333 0.3125 0.31666667 0.32083333 0.325 0.32916667 0.33333333 0.3375 0.34166667 0.34583333 0.35 0.35416667 0.35833333 0.3625 0.36666667 0.37083333 0.375 0.37916667 0.38333333 0.3875 0.39166667 0.39583333 0.4 0.40416667 0.40833333 0.4125 0.41666667 0.42083333 0.425 0.42916667 0.43333333 0.4375 0.44166667 0.44583333 0.45 0.45416667 0.45833333 0.4625 0.46666667 0.47083333 0.475 0.47916667 0.48333333 0.4875 0.49166667 0.49583333 0.5 0.50416667 0.50833333 0.5125 0.51666667 0.52083333 0.525 0.52916667 0.53333333 0.5375 0.54166667 0.54583333 0.55 0.55416667 0.55833333 0.5625 0.56666667 0.57083333 0.575 0.57916667 0.58333333 0.5875 0.59166667 0.59583333 0.6 0.60416667 0.60833333 0.6125 0.61666667 0.62083333 0.625 0.62916667 0.63333333 0.6375 0.64166667 0.64583333 0.65 0.65416667 0.65833333 0.6625 0.66666667 0.67083333 0.675 0.67916667 0.68333333 0.6875 0.69166667 0.69583333 0.7 0.70416667 0.70833333 0.7125 0.71666667 0.72083333 0.725 0.72916667 0.73333333 0.7375 0.74166667 0.74583333 0.75 0.75416667 0.75833333 0.7625 0.76666667 0.77083333 0.775 0.77916667 0.78333333 0.7875 0.79166667 0.79583333 0.8 0.80416667 0.80833333 0.8125 0.81666667 0.82083333 0.825 0.82916667 0.83333333 0.8375 0.84166667 0.84583333 0.85 0.85416667 0.85833333 0.8625 0.86666667 0.87083333 0.875 0.87916667 0.88333333 0.8875 0.89166667 0.89583333 0.9 0.90416667 0.90833333 0.9125 0.91666667 0.92083333 0.925 0.92916667 0.93333333 0.9375 0.94166667 0.94583333 0.95 0.95416667 0.95833333 0.9625 0.96666667 0.97083333 0.975 0.97916667 0.98333333 0.9875 0.99166667 0.99583333 1 1 1 1 1 1
  arc A27 (0.5405, -9.4846) -> (1.2115, -9.4224) centre (0, 0) ccw